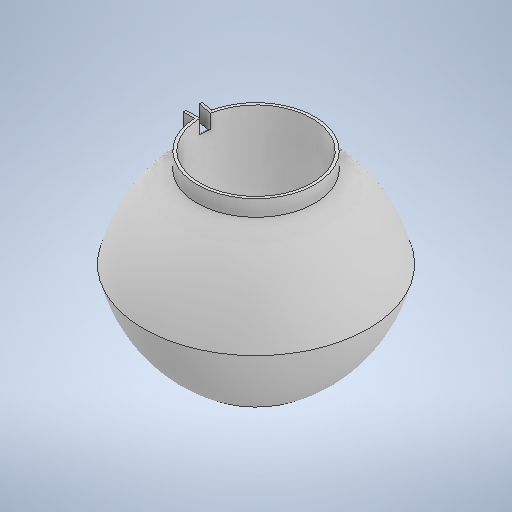
# Autodesk Inventor part: Water Sensor Bouy
Saved by Autodesk Inventor 2025 (Build 290162000, 162)
## iProperties
Created: 2024-06-17
Part Number: Water Sensor Bouy
Material: Generic
Document SubType Name: Modeling
Designer: track
Density: 1 g/cm^3
Appearance: Default
Mass: 1114.84 g
Surface Area: 2537.18 cm^2
Volume: 1114.84 cm^3
Author: track
## iProperties of the stored document Water Sensor Bouy_3DPrint.ipt
Created: 2024-06-17
Part Number: Water Sensor Bouy_3DPrint
Material: Generic
Document SubType Name: Modeling
Designer: track
Density: 1 g/cm^3
Appearance: Default
Author: track
Autodesk Inventor part; units mm, degrees
ref_plane "YZ Plane" through (0, 0, 0) normal (1, 0, 0) x (0, 1, 0)
ref_plane "XZ Plane" through (0, 0, 0) normal (0, 1, 0) x (-1, 0, 0)
ref_plane "XY Plane" through (0, 0, 0) normal (0, 0, 1) x (1, 0, 0)
sketch "Sketch1" plane through (0, 0, 0) normal (0, 0, 1) x (1, 0, 0)
  line L0 (0, 0) -> (0, 76.2)
  line L1 (50.7, 0) -> (50.7, 152.4)
  line L2 (50.7, 76.2) -> (101.5, 76.2)
  arc A0 (101.5, 76.2) -> (50.7, 152.4) centre (-22.4628, 48.5915) ccw
  arc A1 (50.7, 0) -> (101.5, 76.2) centre (-22.4628, 103.8085) ccw
  line L3 (60.7, 130.8894) -> (60.7, 21.5106)
  arc A2 (60.7, 21.5106) -> (91.2332, 76.2) centre (-22.4628, 103.8085) ccw
  arc A3 (91.2332, 76.2) -> (60.7, 130.8894) centre (-22.4628, 48.5915) ccw
  point P0 (50.7, 50.8)
  dimension "d1" = 50.7
  dimension "d3" = 0
  dimension "d74" = 152.4
  dimension "d75" = 50.8
  dimension "d76" = 76.2
  dimension "d78" = 127
  dimension "d83" = 10
  constraints: 8 end point, 8 point on circle, 4 centre point, 2 vertical, 1 horizontal, 1 midpoint, 1 point on line, 3 other
  measures "d1" distance between parallel lines of L1 L0
  measures "d3" vertical distance of L0.start L1.start
  measures "d74" distance of L1.start L1.end
  measures "d75" distance of L2.start L2.end
  measures "d76" distance from line of L1.end L2
  measures "d78" radius of A0
  measures "d83" distance between parallel lines of L1 L3
revolve "Revolution1" add sketch "Sketch1" angle 360 about axis through (0, 0, 0) along (0, 1, 0) contours L1 L2 L3 A2 A1 | L1 A0 L2 A3 L3
sketch "Sketch13" plane through (0, 0, 0) normal (0, 0, 1) x (1, 0, 0)
  line L0 (50.7, 152.4) -> (-50.7, 152.4) projected
  line L1 (0, 152.4) -> (0, 180.8136)
  line L2 (-50.7, 152.4) -> (-50.7, 165.1)
  line L3 (-50.7, 165.1) -> (-53.24, 165.1)
  line L4 (-53.24, 165.1) -> (-53.24, 150.5625)
  arc A0 (-50.7, 152.4) -> (-101.5, 76.2) centre (22.4628, 48.5915) ccw projected
  arc A1 (-50.7, 152.4) -> (-53.24, 150.5625) centre (22.4628, 48.5915) ccw
  point P0 (0, 0)
  dimension "d79" = 2.54
  dimension "d81" = 12.7
  constraints: 8 end point, 3 point on circle, 2 perpendicular, 2 vertical, 1 centre point, 1 concentric, 1 midpoint
  measures "d79" distance of L2.end L3.end
  measures "d81" distance of L0.end L2.end
revolve "Revolution2" add sketch "Sketch13" angle 350 about axis through (0, 152.4, 0) along (0, 1, 0)
sketch "Sketch14" plane through (-52.4312, 150.5625, -9.245) normal (-0.1736482, 0, 0.9848078) x (0.9848078, 0, 0.1736482)
  arc A0 (2.54, 1.8375) -> (0, 0) centre (75.7028, -101.971) ccw projected
  line L0 (0, 0) -> (-10.16, 0)
  line L1 (2.54, 1.8375) -> (2.54, 14.5375) projected
  line L2 (2.54, 14.5375) -> (-10.16, 14.5375)
  line L3 (-10.16, 14.5375) -> (-10.16, 0)
  line L4 (0, 14.5375) -> (0, 0) projected
  line L5 (0, 0) -> (2.54, 1.8375)
  line L6 (2.54, 1.8375) -> (2.54, 14.5375)
  line L7 (0.8088, 14.5375) -> (0.8088, 0) projected
  point P0 (53.24, -150.5625)
  dimension "d84" = 12.7
  dimension "d85" = 14.5375
  constraints: 10 end point, 2 horizontal, 2 parallel
  measures "d84" distance of L1.end L2.end
  measures "d85" distance of L2.end L0.end
extrude "Extrusion8" add sketch "Sketch14" against normal blind 2.54 contours A0 L7 L2 L1 | A0 L4 L2 L7 | L0 L3 L2 L4
sketch "Sketch15" plane through (-50.7, 165.1, 0) normal (0, 0, -1) x (-1, 0, 0)
  arc A0 (2.54, -14.5375) -> (0, -12.7) centre (-73.1628, -116.5085) ccw projected
  line L0 (0, -12.7) -> (2.54, -14.5375)
  line L1 (2.54, -14.5375) -> (12.7, -14.5375)
  line L2 (10, -143.5894) -> (10, -34.2106) projected
  line L3 (0, 0) -> (2.54, 0) projected
  line L4 (0, -12.7) -> (0, 0)
  line L5 (0, 0) -> (12.7, 0)
  line L6 (12.7, 0) -> (12.7, -14.5375)
  point P0 (-50.7, -165.1)
  dimension "d88" = 12.7
  constraints: 10 end point, 4 perpendicular
  measures "d88" distance of L3.start L5.end
extrude "Extrusion9" add sketch "Sketch15" against normal blind 2.54 contours A0 L4 L3 L5 L6 L1
sketch "Sketch16" plane through (-50.7, 165.1, 2.54) normal (0, 0, 1) x (1, 0, 0)
  point P0 (50.7, -165.1)
body "Solid1"
